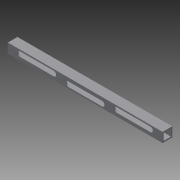
# Autodesk Inventor part: West Coast Side
Saved by Autodesk Inventor 2013 (Build 170138000, 138)
## iProperties
Created: 2014-08-13
Part Number: West Coast Side
Material: Generic
Document SubType Name: Modeling
Designer: kahohbein
Density: 1 g/cm^3
Author: kahohbein
Autodesk Inventor part; units mm, degrees
ref_plane "YZ Plane" through (0, 0, 0) normal (1, 0, 0) x (0, 1, 0)
ref_plane "XZ Plane" through (0, 0, 0) normal (0, 1, 0) x (-1, 0, 0)
ref_plane "XY Plane" through (0, 0, 0) normal (0, 0, 1) x (1, 0, 0)
sketch "Sketch1" plane through (0, 0, 0) normal (0, 0, 1) x (1, 0, 0)
  line L0 (0, 0) -> (406.4, 0)
  line L1 (406.4, 0) -> (406.4, 25.4)
  line L2 (406.4, 25.4) -> (0, 25.4)
  line L3 (0, 25.4) -> (0, 0)
  dimension "d0" = 406.4
  dimension "d1" = 25.4
  constraints: 8 end point, 2 parallel, 1 horizontal, 1 perpendicular
  measures "d0" distance of L2.end L1.end
  measures "d1" distance of L1.end L0.end
extrude "Extrusion1" add sketch "Sketch1" along normal blind 25.4
sketch "Sketch2" plane through (406.4, 0, 0) normal (1, 0, 0) x (0, 0, -1)
  line L0 (-22.225, 3.4845) -> (-3.175, 3.4845)
  line L1 (-3.175, 3.4845) -> (-3.175, 21.9155)
  line L2 (-3.175, 21.9155) -> (-22.225, 21.9155)
  line L3 (-22.225, 21.9155) -> (-22.225, 3.4845)
  line L4 (-22.225, 3.4845) -> (-3.175, 21.9155) construction
  line L5 (-3.175, 3.4845) -> (-22.225, 21.9155) construction
  point P0 (-12.7, 12.7)
  dimension "d4" = 19.05
  constraints: 12 end point, 2 midpoint, 2 parallel, 1 horizontal, 1 perpendicular
  measures "d4" distance of L2.end L1.end
extrude "Extrusion2" cut sketch "Sketch2" against normal blind 406.4
sketch "Sketch3" plane through (0, 0, 25.4) normal (0, 0, 1) x (1, 0, 0)
  arc A0 (31.75, 21.59) -> (31.75, 8.89) centre (31.75, 15.24) ccw
  arc A1 (120.65, 8.89) -> (120.65, 21.59) centre (120.65, 15.24) ccw
  line L0 (31.75, 21.59) -> (120.65, 21.59)
  line L1 (31.75, 8.89) -> (120.65, 8.89)
  arc A2 (158.75, 16.51) -> (158.75, 3.81) centre (158.75, 10.16) ccw
  arc A3 (247.65, 3.81) -> (247.65, 16.51) centre (247.65, 10.16) ccw
  line L2 (158.75, 16.51) -> (247.65, 16.51)
  line L3 (247.65, 3.81) -> (158.75, 3.81)
  line L4 (0, 0) -> (406.4, 0) projected
  line L5 (406.4, 25.4) -> (0, 25.4) projected
  line L6 (0, 25.4) -> (0, 0) projected
  line L7 (25.4, 15.24) -> (25.4, 25.4)
  line L8 (127, 15.24) -> (127, 25.4)
  line L9 (152.4, 10.16) -> (152.4, 0)
  line L10 (254, 10.16) -> (254, 0)
  arc A4 (285.75, 21.59) -> (285.75, 8.89) centre (285.75, 15.24) ccw
  arc A5 (374.65, 8.89) -> (374.65, 21.59) centre (374.65, 15.24) ccw
  line L11 (279.4, 15.24) -> (279.4, 25.4)
  line L12 (285.75, 21.59) -> (374.65, 21.59)
  line L13 (381, 15.24) -> (381, 25.4)
  line L14 (374.65, 8.89) -> (285.75, 8.89)
  line L15 (158.75, 0) -> (158.75, 10.16)
  line L16 (31.75, 15.24) -> (31.75, 25.4)
  line L17 (374.65, 15.24) -> (374.65, 25.4)
  dimension "d7" = 12.7
  dimension "d8" = 12.7
  dimension "d13" = 12.7
  dimension "d14" = 12.7
  dimension "d19" = 101.6
  dimension "d20" = 101.6
  dimension "d22" = 12.7
  dimension "d23" = 12.7
  dimension "d24" = 101.6
  dimension "d25" = 25.4
  dimension "d26" = 25.4
  dimension "d27" = 25.4
  dimension "d28" = 10.16
  dimension "d29" = 10.16
  constraints: 30 end point, 18 point on circle, 12 tangent, 10 point on line, 6 centre point, 5 parallel, 5 perpendicular
  measures "d7" diameter of A0
  measures "d8" diameter of A1
  measures "d13" diameter of A2
  measures "d14" diameter of A3
  measures "d19" distance between parallel lines of L8 L7
  measures "d20" distance between parallel lines of L10 L9
  measures "d22" diameter of A4
  measures "d23" diameter of A5
  measures "d24" distance between parallel lines of L13 L11
  measures "d25" distance between parallel lines of L7 L6
  measures "d26" distance between parallel lines of L9 L8
  measures "d27" distance between parallel lines of L10 L11
  measures "d28" distance of L15.start L15.end
  measures "d29" distance of L16.start L16.end
extrude "Extrusion3" cut sketch "Sketch3" against normal blind 25.4 contours L0 A1 L1 A0 | A4 L12 A5 L14 | A2 L2 A3 L3
body "Solid1"
